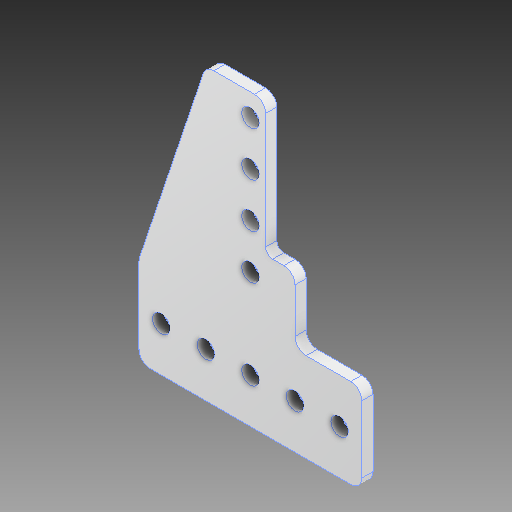
# Autodesk Inventor part: Elevator Mounting Gusset
Saved by Autodesk Inventor 2022 (Build 260153000, 153)
## iProperties
Created: 2020-09-05
Part Number: Elevator Mounting Gusset
Material: Aluminum 6061
Document SubType Name: Modeling
Density: 2.7 g/cm^3
Appearance: Aluminum - Flat
Autodesk Inventor part; units mm, degrees
ref_plane "YZ Plane" through (0, 0, 0) normal (1, 0, 0) x (0, 1, 0)
ref_plane "XZ Plane" through (0, 0, 0) normal (0, 1, 0) x (-1, 0, 0)
ref_plane "XY Plane" through (0, 0, 0) normal (0, 0, 1) x (1, 0, 0)
sketch "Sketch1" plane through (0, 0, 0) normal (0, 0, 1) x (1, 0, 0)
  circle A0 centre (-12.7, 12.7) radius 2.4892
  line L0 (19.05, 0) -> (-44.45, 0)
  line L1 (-44.45, 0) -> (-44.45, -25.4)
  line L2 (-44.45, -25.4) -> (19.05, -25.4)
  line L3 (19.05, -25.4) -> (19.05, 0)
  line L4 (19.05, 0) -> (-44.45, -25.4) construction
  line L5 (-44.45, 0) -> (19.05, -25.4) construction
  line L6 (0, 57.15) -> (-25.4, 57.15)
  line L7 (-25.4, 57.15) -> (-25.4, 0)
  line L8 (-25.4, 0) -> (0, 0)
  line L9 (0, 0) -> (0, 57.15)
  line L10 (0, 57.15) -> (-25.4, 0) construction
  line L11 (-25.4, 57.15) -> (0, 0) construction
  line L12 (-25.4, 57.15) -> (-44.45, 0)
  circle A1 centre (-12.7, 25.4) radius 2.4892
  circle A2 centre (-12.7, 38.1) radius 2.4892
  circle A3 centre (-12.7, 50.8) radius 2.4892
  circle A4 centre (-38.1, -12.7) radius 2.4892
  circle A5 centre (-25.4, -12.7) radius 2.4892
  circle A6 centre (-12.7, -12.7) radius 2.4892
  circle A7 centre (0, -12.7) radius 2.4892
  circle A8 centre (12.7, -12.7) radius 2.4892
  line L13 (0, 57.15) -> (-8.382, 57.15)
  line L14 (-8.382, 57.15) -> (-8.382, 19.05)
  line L15 (-8.382, 19.05) -> (0, 19.05)
  line L16 (0, 19.05) -> (0, 57.15)
  point P0 (0, 0)
  point P1 (-12.7, -12.7)
  point P2 (-12.7, 28.575)
  point P3 (-12.7, 57.15)
  point P4 (-44.45, -12.7)
  point P5 (0, 19.05)
  dimension "d0" = 4.9784
  dimension "d1" = 25.4
  dimension "d2" = 25.4
  dimension "d5" = 12.7
  dimension "d10" = 6.35
  dimension "d11" = 12.7
  dimension "d12" = 19.05
  dimension "d15" = 12.7
  dimension "d21" = 6.35
  dimension "d25" = 8.382
  dimension "d26" = 6.35
  dimension "d28" = 6.35
  constraints: 34 end point, 9 centre point, 6 midpoint, 6 parallel, 4 horizontal, 3 perpendicular, 1 coincident, 1 equal radius, 1 horizontal alignment, 1 point on line, 1 vertical, 1 vertical alignment, 14 other
  measures "d0" diameter of A0
  measures "d1" distance of L1.end L0.end
  measures "d2" distance of L8.end L7.end
  measures "d5" distance of A0.centre A1.centre
  measures "d10" distance from line of L6 A3.centre
  measures "d11" distance from line of L8 A0.centre
  measures "d12" distance between parallel lines of L1 L7
  measures "d15" distance of A4.centre A5.centre
  measures "d21" distance from line of L1 A4.centre
  measures "d25" distance of L15.end L14.end
  measures "d26" distance from line of A0.centre L15
  measures "d28" distance from line of L3 A8.centre
extrude "Extrusion1" add sketch "Sketch1" along normal blind 3.175 contours L3 L2 L1 L0 | L0 L7 L6 L14 L15 L9 | L0 L12 L7
fillet "Fillet1" radius 3.175 8 edges at (19.05, 0, 1.5875) (19.05, -25.4, 1.5875) (-44.45, -25.4, 1.5875) (0, 0, 1.5875) (-44.45, 0, 1.5875) (-25.4, 57.15, 1.5875) (-8.382, 57.15, 1.5875) (0, 19.05, 1.5875)
fillet "Fillet1" radius 2 1 edges at (-8.382, 19.05, 1.5875)
equation "\"d28\" = d21"
body "Solid1"
